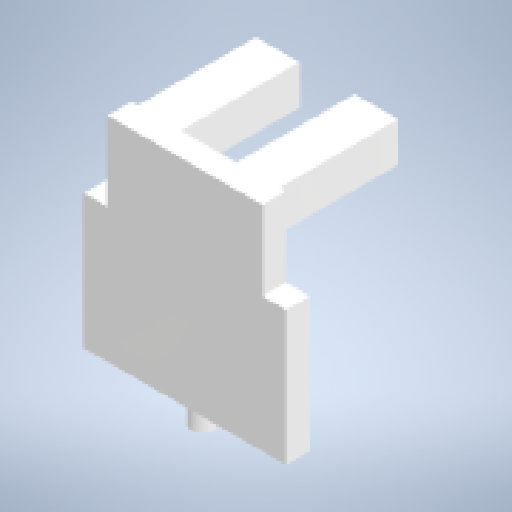
# Autodesk Inventor part: SchubstangeA
Saved by Autodesk Inventor 2025 (Build 290162010, 162A)
## iProperties
Created: 2024-11-26
Part Number: SchubstangeA
Material: PC/ABS-Kunststoff, 3DDruck, PLA
Document SubType Name: Modeling
Designer: Admin
Density: 1.1 g/cm^3
Appearance: Glatt - Weiß(2)
Author: Admin
Autodesk Inventor part; units mm, degrees
ref_plane "YZ Plane" through (0, 0, 0) normal (1, 0, 0) x (0, 1, 0)
ref_plane "XZ Plane" through (0, 0, 0) normal (0, 1, 0) x (-1, 0, 0)
ref_plane "XY Plane" through (0, 0, 0) normal (0, 0, 1) x (1, 0, 0)
sketch "Skizze1" plane through (0, 0, 0) normal (0, 1, 0) x (-1, 0, 0)
  line L0 (16.6592, -116.2444) -> (-8.9408, -116.2444)
  line L1 (-8.9408, -116.2444) -> (-8.9408, -89.2444)
  line L2 (16.6592, -89.2444) -> (16.6592, -116.2444)
  line L3 (3.8592, 157.3916) -> (3.8592, -262.6084)
  line L4 (16.6592, -89.2444) -> (-8.9408, -89.2444)
  line L5 (-8.9408, -89.2444) -> (-5.9408, -89.2444)
  line L6 (-5.9408, -89.2444) -> (-5.9408, -99.2444)
  line L7 (-5.9408, -99.2444) -> (-8.9408, -99.2444)
  line L8 (-8.9408, -99.2444) -> (-8.9408, -89.2444)
  line L9 (16.6592, -89.2444) -> (13.6592, -89.2444)
  line L10 (13.6592, -89.2444) -> (13.6592, -99.2444)
  line L11 (13.6592, -99.2444) -> (16.6592, -99.2444)
  line L12 (16.6592, -99.2444) -> (16.6592, -89.2444)
  point P0 (0, 0)
  point P1 (3.8592, -116.2444)
  point P2 (16.6592, -99.2444)
  point P3 (13.6592, -89.2444)
  dimension "d1" = 27
  dimension "d9" = 25.6
  dimension "d56" = 3
  dimension "d57" = 10
  dimension "d58" = 3
  dimension "d59" = 10
  constraints: 26 end point, 5 horizontal, 5 parallel, 3 perpendicular, 1 midpoint, 1 point on line, 1 vertical, 2 other
  measures "d1" distance of L0.end L1.end
  measures "d9" distance of L0.start L0.end
  measures "d56" distance of L6.end L7.end
  measures "d57" distance of L5.end L6.end
  measures "d58" distance of L11.end L10.end
  measures "d59" distance of L10.end L9.end
extrude "Extrusion1" add sketch "Skizze1" along normal blind 3 contours L0 L3 L4 L10 L11 L2 | L0 L1 L7 L6 L4 L3
sketch "Skizze3" plane through (0.1408, 0, -116.2444) normal (0, 0, -1) x (-1, 0, 0)
  line L0 (-3.8, 0) -> (-3.8, 3.3)
  circle A0 centre (-3.8, 3.3) radius 2.5
  line L1 (16.8, 0) -> (-8.8, 0)
  line L2 (-8.8, 0) -> (16.8, 0) projected
  line L3 (11.8, 0) -> (11.8, 3.3)
  circle A1 centre (11.8, 3.3) radius 2.5
  dimension "d29" = 5
  dimension "d60" = 5
  dimension "d61" = 3.3
  dimension "d62" = 5
  dimension "d63" = 3.3
  dimension "d64" = 5
  constraints: 8 end point, 2 centre point, 2 point on line, 2 vertical, 1 horizontal, 2 other
  measures "d29" diameter of A0
  measures "d60" distance from line of L1.end L0
  measures "d61" distance of L0.start L0.end
  measures "d62" diameter of A1
  measures "d63" distance of L3.start L3.end
  measures "d64" horizontal distance of L1.start L3.end
extrude "Extrusion2" add sketch "Skizze3" along normal blind 4
sketch "Skizze5" plane through (0, 3, 0) normal (0, 1, 0) x (1, 0, 0)
  line L0 (5.1408, 89.2444) -> (-12.8592, 89.2444)
  line L1 (-12.8592, 94.2444) -> (5.1408, 94.2444)
  line L2 (5.1408, 94.2444) -> (5.1408, 89.2444)
  line L3 (-7.3592, 89.2444) -> (-0.3592, 89.2444)
  line L4 (-0.3592, 89.2444) -> (-0.3592, 94.2444)
  line L5 (-0.3592, 94.2444) -> (-7.3592, 94.2444)
  line L6 (-7.3592, 94.2444) -> (-7.3592, 89.2444)
  line L7 (-7.3592, 91.7444) -> (-12.8592, 91.7444) construction
  line L8 (-0.3592, 91.7444) -> (5.1408, 91.7444) construction
  line L9 (-12.8592, 94.2444) -> (-12.8592, 89.2444)
  line L10 (-13.6592, 89.2444) -> (5.9408, 89.2444) projected
  point P0 (0, 0)
  point P1 (-0.3592, 89.2444)
  point P2 (-7.3592, 94.2444)
  point P3 (-16.6592, 86.2444)
  point P4 (8.9408, 86.2444)
  point P5 (-3.8592, 89.2444)
  point P6 (5.9408, 89.2444)
  dimension "d43" = 7
  dimension "d54" = 5
  dimension "d55" = 18
  constraints: 20 end point, 5 midpoint, 4 parallel, 3 horizontal, 2 coincident, 2 point on line, 1 collinear, 1 perpendicular, 1 vertical, 2 other
  measures "d43" distance between parallel lines of L6 L4
  measures "d54" distance between parallel lines of L0 L1
  measures "d55" distance between parallel lines of L2 L9
extrude "Extrusion4" add sketch "Skizze5" along normal blind 10 contours L0 L4 L1 L2 | L0 L9 L1 L6
sketch "Skizze6" plane through (0, 3, 0) normal (0, 1, 0) x (1, 0, 0)
  line L0 (8.9408, 116.2444) -> (-16.6592, 116.2444) projected
  line L1 (7.4408, 116.2444) -> (0.4408, 116.2444)
  line L2 (0.4408, 116.2444) -> (0.4408, 115.2444)
  line L3 (0.4408, 115.2444) -> (7.4408, 115.2444)
  line L4 (7.4408, 115.2444) -> (7.4408, 116.2444)
  line L5 (-15.1592, 116.2444) -> (-8.1592, 116.2444)
  line L6 (-8.1592, 116.2444) -> (-8.1592, 115.2444)
  line L7 (-8.1592, 115.2444) -> (-15.1592, 115.2444)
  line L8 (-15.1592, 115.2444) -> (-15.1592, 116.2444)
  line L9 (6.4408, 116.2444) -> (1.4408, 116.2444) projected
  line L10 (-9.1592, 116.2444) -> (-14.1592, 116.2444) projected
  point P0 (0, 0)
  point P1 (1.4589, 116.2444)
  point P2 (6.4227, 116.2444)
  point P3 (-14.1411, 116.2444)
  point P4 (-9.1773, 116.2444)
  point P5 (3.9408, 116.2444)
  point P6 (-11.6592, 116.2444)
  point P7 (-8.1592, 116.2444)
  point P8 (-15.1592, 116.2444)
  point P9 (0.4408, 116.2444)
  dimension "d65" = 7
  dimension "d66" = 1
  dimension "d67" = 7
  dimension "d68" = 1
  constraints: 16 end point, 4 midpoint, 4 parallel, 2 horizontal, 2 perpendicular, 1 point on line, 2 other
  measures "d65" distance of L3.end L2.end
  measures "d66" distance of L2.end L1.end
  measures "d67" distance of L7.end L6.end
  measures "d68" distance of L6.end L5.end
extrude "Extrusion5" add sketch "Skizze6" along normal blind 4
